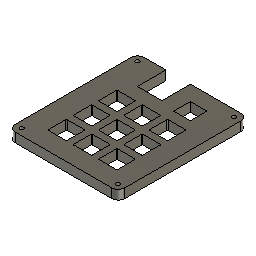
prvpad_top (Autodesk Fusion 360 design; units mm, degrees)
part number: 2026-03-06-21-55-46-293
Autodesk Fusion 360 part; units mm, degrees
sketch "Sketch1" plane through (0, 0, 0) normal (0, 0, 1) x (1, 0, 0)
  line L0 (40.8554, 59.6943) -> (40.8554, -37.5959)
  line L1 (-41.8946, 59.6943) -> (40.8554, 59.6943)
  line L2 (-41.8946, -37.5959) -> (-41.8946, 59.6943)
  line L3 (40.8554, -37.5959) -> (-41.8946, -37.5959)
  line L4 (-25.4246, 28.1391) -> (-12.4246, 28.1391)
  line L5 (-25.4246, 14.1391) -> (-12.4246, 14.1391)
  line L6 (-25.9246, 27.6391) -> (-25.9246, 14.6391)
  line L7 (-11.9246, 27.6391) -> (-11.9246, 14.6391)
  arc A0 (-25.4246, 28.1391) -> (-25.9246, 27.6391) centre (-25.4246, 27.6391) ccw
  arc A1 (-11.9246, 27.6391) -> (-12.4246, 28.1391) centre (-12.4246, 27.6391) ccw
  arc A2 (-25.9246, 14.6391) -> (-25.4246, 14.1391) centre (-25.4246, 14.6391) ccw
  arc A3 (-12.4246, 14.1391) -> (-11.9246, 14.6391) centre (-12.4246, 14.6391) ccw
  line L8 (-6.3746, 28.1391) -> (6.6254, 28.1391)
  line L9 (-6.3746, 14.1391) -> (6.6254, 14.1391)
  line L10 (-6.8746, 27.6391) -> (-6.8746, 14.6391)
  line L11 (7.1254, 27.6391) -> (7.1254, 14.6391)
  arc A4 (-6.3746, 28.1391) -> (-6.8746, 27.6391) centre (-6.3746, 27.6391) ccw
  arc A5 (7.1254, 27.6391) -> (6.6254, 28.1391) centre (6.6254, 27.6391) ccw
  arc A6 (-6.8746, 14.6391) -> (-6.3746, 14.1391) centre (-6.3746, 14.6391) ccw
  arc A7 (6.6254, 14.1391) -> (7.1254, 14.6391) centre (6.6254, 14.6391) ccw
  line L12 (12.6754, 28.1391) -> (25.6754, 28.1391)
  line L13 (12.6754, 14.1391) -> (25.6754, 14.1391)
  line L14 (12.1754, 27.6391) -> (12.1754, 14.6391)
  line L15 (26.1754, 27.6391) -> (26.1754, 14.6391)
  arc A8 (12.6754, 28.1391) -> (12.1754, 27.6391) centre (12.6754, 27.6391) ccw
  arc A9 (26.1754, 27.6391) -> (25.6754, 28.1391) centre (25.6754, 27.6391) ccw
  arc A10 (12.1754, 14.6391) -> (12.6754, 14.1391) centre (12.6754, 14.6391) ccw
  arc A11 (25.6754, 14.1391) -> (26.1754, 14.6391) centre (25.6754, 14.6391) ccw
  line L16 (-25.4246, 9.0891) -> (-12.4246, 9.0891)
  line L17 (-25.4246, -4.9109) -> (-12.4246, -4.9109)
  line L18 (-25.9246, 8.5891) -> (-25.9246, -4.4109)
  line L19 (-11.9246, 8.5891) -> (-11.9246, -4.4109)
  arc A12 (-25.4246, 9.0891) -> (-25.9246, 8.5891) centre (-25.4246, 8.5891) ccw
  arc A13 (-11.9246, 8.5891) -> (-12.4246, 9.0891) centre (-12.4246, 8.5891) ccw
  arc A14 (-25.9246, -4.4109) -> (-25.4246, -4.9109) centre (-25.4246, -4.4109) ccw
  arc A15 (-12.4246, -4.9109) -> (-11.9246, -4.4109) centre (-12.4246, -4.4109) ccw
  line L20 (-6.3746, 9.0891) -> (6.6254, 9.0891)
  line L21 (-6.3746, -4.9109) -> (6.6254, -4.9109)
  line L22 (-6.8746, 8.5891) -> (-6.8746, -4.4109)
  line L23 (7.1254, 8.5891) -> (7.1254, -4.4109)
  arc A16 (-6.3746, 9.0891) -> (-6.8746, 8.5891) centre (-6.3746, 8.5891) ccw
  arc A17 (7.1254, 8.5891) -> (6.6254, 9.0891) centre (6.6254, 8.5891) ccw
  arc A18 (-6.8746, -4.4109) -> (-6.3746, -4.9109) centre (-6.3746, -4.4109) ccw
  arc A19 (6.6254, -4.9109) -> (7.1254, -4.4109) centre (6.6254, -4.4109) ccw
  line L24 (12.6754, 9.0891) -> (25.6754, 9.0891)
  line L25 (12.6754, -4.9109) -> (25.6754, -4.9109)
  line L26 (12.1754, 8.5891) -> (12.1754, -4.4109)
  line L27 (26.1754, 8.5891) -> (26.1754, -4.4109)
  arc A20 (12.6754, 9.0891) -> (12.1754, 8.5891) centre (12.6754, 8.5891) ccw
  arc A21 (26.1754, 8.5891) -> (25.6754, 9.0891) centre (25.6754, 8.5891) ccw
  arc A22 (12.1754, -4.4109) -> (12.6754, -4.9109) centre (12.6754, -4.4109) ccw
  arc A23 (25.6754, -4.9109) -> (26.1754, -4.4109) centre (25.6754, -4.4109) ccw
  line L28 (-25.4246, -9.9609) -> (-12.4246, -9.9609)
  line L29 (-25.4246, -23.9609) -> (-12.4246, -23.9609)
  line L30 (-25.9246, -10.4609) -> (-25.9246, -23.4609)
  line L31 (-11.9246, -10.4609) -> (-11.9246, -23.4609)
  arc A24 (-25.4246, -9.9609) -> (-25.9246, -10.4609) centre (-25.4246, -10.4609) ccw
  arc A25 (-11.9246, -10.4609) -> (-12.4246, -9.9609) centre (-12.4246, -10.4609) ccw
  arc A26 (-25.9246, -23.4609) -> (-25.4246, -23.9609) centre (-25.4246, -23.4609) ccw
  arc A27 (-12.4246, -23.9609) -> (-11.9246, -23.4609) centre (-12.4246, -23.4609) ccw
  line L32 (-6.3746, -9.9609) -> (6.6254, -9.9609)
  line L33 (-6.3746, -23.9609) -> (6.6254, -23.9609)
  line L34 (-6.8746, -10.4609) -> (-6.8746, -23.4609)
  line L35 (7.1254, -10.4609) -> (7.1254, -23.4609)
  arc A28 (-6.3746, -9.9609) -> (-6.8746, -10.4609) centre (-6.3746, -10.4609) ccw
  arc A29 (7.1254, -10.4609) -> (6.6254, -9.9609) centre (6.6254, -10.4609) ccw
  arc A30 (-6.8746, -23.4609) -> (-6.3746, -23.9609) centre (-6.3746, -23.4609) ccw
  arc A31 (6.6254, -23.9609) -> (7.1254, -23.4609) centre (6.6254, -23.4609) ccw
  line L36 (12.6754, -9.9609) -> (25.6754, -9.9609)
  line L37 (12.6754, -23.9609) -> (25.6754, -23.9609)
  line L38 (12.1754, -10.4609) -> (12.1754, -23.4609)
  line L39 (26.1754, -10.4609) -> (26.1754, -23.4609)
  arc A32 (12.6754, -9.9609) -> (12.1754, -10.4609) centre (12.6754, -10.4609) ccw
  arc A33 (26.1754, -10.4609) -> (25.6754, -9.9609) centre (25.6754, -10.4609) ccw
  arc A34 (12.1754, -23.4609) -> (12.6754, -23.9609) centre (12.6754, -23.4609) ccw
  arc A35 (25.6754, -23.9609) -> (26.1754, -23.4609) centre (25.6754, -23.4609) ccw
  line L40 (9.2304, 48.2841) -> (21.7304, 48.2841)
  line L41 (21.7304, 48.2841) -> (21.7304, 35.7841)
  line L42 (21.7304, 35.7841) -> (9.2304, 35.7841)
  line L43 (9.2304, 35.7841) -> (9.2304, 48.2841)
  line L44 (-20.5696, 59.6943) -> (-2.0696, 59.6943)
  line L45 (-2.0696, 59.6943) -> (-2.0696, 38.1943)
  line L46 (-2.0696, 38.1943) -> (-20.5696, 38.1943)
  line L47 (-20.5696, 38.1943) -> (-20.5696, 59.6943)
  circle A36 centre (-36.8946, 54.6943) radius 1.45
  circle A37 centre (35.8554, 54.6943) radius 1.45
  circle A38 centre (35.8554, -32.5959) radius 1.45
  circle A39 centre (-36.8946, -32.5959) radius 1.45
  dimension "d1" = 14.68
  dimension "d2" = 13.635
  dimension "d3" = 12.5
  dimension "d4" = 12.5
  dimension "d5" = 19.125
  dimension "d6" = 7.645
  dimension "d7" = 18.5
  dimension "d8" = 21.5
  dimension "d9" = 11.3
  dimension "d10" = 2.9
  dimension "d11" = 5
  dimension "d12" = 5
  dimension "d13" = 2.9
  dimension "d14" = 5
  dimension "d15" = 5
  dimension "d16" = 2.9
  dimension "d17" = 5
  dimension "d18" = 5
  dimension "d19" = 2.9
  dimension "d20" = 5
  dimension "d21" = 5
  constraint horizontal L1
  constraint vertical L0
  constraint horizontal L3
  constraint vertical L2
  constraint horizontal L40
  constraint vertical L41
  constraint horizontal L42
  constraint vertical L43
  constraint horizontal L44
  constraint vertical L45
  constraint horizontal L46
  constraint vertical L47
  constraint coincident L1 L44.start
  measures "d1" distance of L0 L39
  measures "d2" distance of L3 L37
  measures "d3" distance of L40 L42
  measures "d4" distance of L41 L43
  measures "d5" distance of L0 L41
  measures "d6" distance of L12 L42
  measures "d7" distance of L45 L47
  measures "d8" distance of L1 L46
  measures "d9" distance of L43 L45
  measures "d10" diameter of A36
  measures "d11" distance of L1 A36.centre
  measures "d12" distance of L2 A36.centre
  measures "d13" diameter of A39
  measures "d14" distance of L3 A39.centre
  measures "d15" distance of L2 A39.centre
  measures "d16" diameter of A38
  measures "d17" distance of L0 A38.centre
  measures "d18" distance of L3 A38.centre
  measures "d19" diameter of A37
  measures "d20" distance of L1 A37.centre
  measures "d21" distance of L0 A37.centre
extrude "Extrude1" add sketch "Sketch1" along normal blind 7 contours L0 L1 L2 L3 L45 L46 L47
fillet "Fillet1" radius 5 4 edges at (-41.8946, 59.6943, 3.5) (-41.8946, -37.5959, 3.5) (40.8554, -37.5959, 3.5) (40.8554, 59.6943, 3.5)
